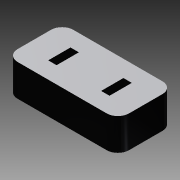
# Autodesk Inventor part: RETAINER
Saved by Autodesk Inventor 2013 (Build 170138000, 138)
## iProperties
Created: 2014-06-21
Part Number: RETAINER
Material: Generic
Document SubType Name: Modeling
Designer: employee
Density: 1 g/cm^3
Author: employee
Autodesk Inventor part; units mm, degrees
ref_plane "YZ Plane" through (0, 0, 0) normal (1, 0, 0) x (0, 1, 0)
ref_plane "XZ Plane" through (0, 0, 0) normal (0, 1, 0) x (-1, 0, 0)
ref_plane "XY Plane" through (0, 0, 0) normal (0, 0, 1) x (1, 0, 0)
sketch "Sketch1" plane through (0, 0, 0) normal (0, 0, 1) x (1, 0, 0)
  line L0 (-10, 5) -> (10, 5)
  line L1 (10, 5) -> (10, -5)
  line L2 (10, -5) -> (-10, -5)
  line L3 (-10, -5) -> (-10, 5)
  line L4 (-5.5, 2) -> (-4, 2)
  line L5 (-4, 2) -> (-4, -2)
  line L6 (-4, -2) -> (-5.5, -2)
  line L7 (-5.5, -2) -> (-5.5, 2)
  line L8 (5.5, 2) -> (4, 2)
  line L9 (4, 2) -> (4, -2)
  line L10 (4, -2) -> (5.5, -2)
  line L11 (5.5, -2) -> (5.5, 2)
  line L12 (-4, 0) -> (4, 0)
  point P0 (0, 0)
  point P1 (-10, 0)
  point P2 (0, 5)
  point P3 (0, 0)
  dimension "d0" = 20
  dimension "d2" = 10
  dimension "d3" = 8
  dimension "d4" = 1.5
  dimension "d5" = 4
  constraints: 26 end point, 6 parallel, 5 midpoint, 4 perpendicular, 3 horizontal, 3 horizontal alignment, 2 equal length, 1 coincident, 1 vertical alignment
  measures "d0" distance of L1.end L2.end
  measures "d2" distance of L0.end L1.end
  measures "d3" distance of L12.start L12.end
  measures "d4" distance of L9.end L10.end
  measures "d5" distance of L10.end L8.start
extrude "Extrusion1" add sketch "Sketch1" along normal blind 5.715
fillet "Fillet1" radius 2 4 edges at (-10, 5, 2.8575) (10, 5, 2.8575) (10, -5, 2.8575) (-10, -5, 2.8575)
body "Solid1"
